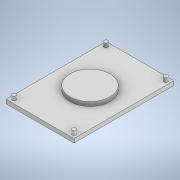
# Autodesk Inventor part: тест
Saved by Autodesk Inventor 2022 (Build 260153000, 153)
## iProperties
Created: 2023-02-28
Part Number: тест
Material: Типовые
Document SubType Name: Modeling
Designer: Папа
Density: 1 g/cm^3
Appearance: По умолчанию
Author: Папа
Autodesk Inventor part; units mm, degrees
ref_plane "YZ Plane" through (0, 0, 0) normal (1, 0, 0) x (0, 1, 0)
ref_plane "XZ Plane" through (0, 0, 0) normal (0, 1, 0) x (-1, 0, 0)
ref_plane "XY Plane" through (0, 0, 0) normal (0, 0, 1) x (1, 0, 0)
sketch "Эскиз1" plane through (0, 0, 0) normal (0, 1, 0) x (-1, 0, 0)
  line L0 (14.899, 13.3523) -> (-2.101, 13.3523)
  line L1 (-2.101, 13.3523) -> (-2.101, -11.6477)
  line L2 (-2.101, -11.6477) -> (14.899, -11.6477)
  line L3 (14.899, -11.6477) -> (14.899, 13.3523)
  point P0 (0, 0)
  dimension "d0" = 25
  dimension "d1" = 17
  constraints: 8 end point, 2 parallel, 1 horizontal, 1 perpendicular
  measures "d0" distance of L2.end L0.start
  measures "d1" distance of L1.end L2.end
extrude "Выдавливание1" add sketch "Эскиз1" along normal blind 1
sketch "Эскиз2" plane through (0, 1, 0) normal (0, 1, 0) x (1, 0, 0)
  line L0 (-14.899, 11.6477) -> (-14.899, -13.3523) construction
  line L1 (2.101, -13.3523) -> (2.101, 11.6477) construction
  line L2 (-14.899, -13.3523) -> (2.101, 11.6477) construction
  line L3 (2.101, 11.6477) -> (-14.899, 11.6477) construction
  line L4 (-14.899, 11.6477) -> (2.101, -13.3523) construction
  line L5 (-13.899, -12.3523) -> (1.101, -12.3523) construction
  line L6 (1.101, -12.3523) -> (1.101, 10.6477) construction
  line L7 (1.101, 10.6477) -> (-13.899, 10.6477) construction
  line L8 (-13.899, 10.6477) -> (-13.899, -12.3523) construction
  line L9 (-13.899, -12.3523) -> (1.101, 10.6477) construction
  line L10 (1.101, -12.3523) -> (-13.899, 10.6477) construction
  circle A0 centre (-13.899, -12.3523) radius 0.5
  circle A1 centre (-13.899, 10.6477) radius 0.5
  circle A2 centre (1.101, 10.6477) radius 0.5
  circle A3 centre (1.101, -12.3523) radius 0.5
  circle A4 centre (-6.399, -0.8523) radius 5
  point P0 (0, 0)
  point P1 (-6.399, -0.8523)
  dimension "d4" = 23
  dimension "d5" = 15
  dimension "d6" = 1
  dimension "d7" = 10
  constraints: 18 end point, 5 centre point, 5 coincident, 3 equal radius, 3 midpoint, 2 parallel, 2 perpendicular, 1 horizontal
  measures "d4" distance of L7.end L5.start
  measures "d5" distance of L6.end L7.end
  measures "d6" diameter of A1
  measures "d7" diameter of A4
extrude "Выдавливание2" add sketch "Эскиз2" along normal blind 1
